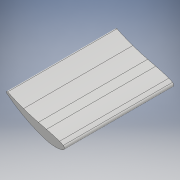
# Autodesk Inventor part: sub flap
Saved by Autodesk Inventor 2018.3 (Build 223284000, 284)
## iProperties
Created: 2018-06-13
Part Number: sub flap
Material: 一般
Document SubType Name: Modeling
Designer: ku_sk
Density: 1 g/cm^3
Appearance: 既定
Author: ku_sk
Autodesk Inventor part; units mm, degrees
ref_plane "YZ Plane" through (0, 0, 0) normal (1, 0, 0) x (0, 1, 0)
ref_plane "XZ Plane" through (0, 0, 0) normal (0, 1, 0) x (-1, 0, 0)
ref_plane "XY Plane" through (0, 0, 0) normal (0, 0, 1) x (1, 0, 0)
sketch "スケッチ1" plane through (0, 0, 0) normal (0, 1, 0) x (-1, 0, 0)
  arc A0 (319.6761, 45.1314) -> (390.0033, 84.5371) centre (233.4832, 281.4189) ccw projected
  arc A1 (390.0033, 84.5371) -> (387.8794, 87.899) centre (388.7587, 86.1027) ccw projected
  arc A2 (355.3068, 74.2795) -> (387.8794, 87.899) centre (256.7374, 355.7795) ccw projected
  arc A3 (324.6713, 65.1488) -> (355.3068, 74.2795) centre (243.2403, 394.3253) ccw projected
  arc A4 (307.9726, 61.0464) -> (324.6713, 65.1488) centre (-955.196, 5238.8807) ccw projected
  arc A5 (307.9726, 61.0464) -> (281.147, 53.127) centre (377.3682, -223.4121) ccw projected
  arc A6 (281.147, 53.127) -> (273.4497, 49.6709) centre (297.0704, 7.3635) ccw projected
  arc A7 (273.4497, 49.6709) -> (273.0796, 42.1444) centre (275.6154, 45.792) ccw projected
  arc A8 (273.0796, 42.1444) -> (277.153, 40.2312) centre (280.7432, 53.1684) ccw projected
  arc A9 (277.153, 40.2312) -> (289.7252, 38.6521) centre (288.8177, 82.2649) ccw projected
  arc A10 (289.7252, 38.6521) -> (309.4937, 41.755) centre (288.1775, 113.0354) ccw projected
  arc A11 (309.4937, 41.755) -> (319.6761, 45.1314) centre (257.566, 215.3987) ccw projected
  point P0 (0, 0)
extrude "押し出し1" add sketch "スケッチ1" along normal blind 225
